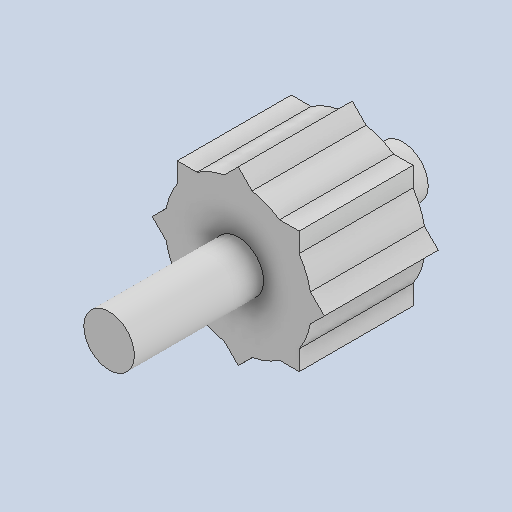
# Autodesk Inventor part: kolo
Saved by Autodesk Inventor 2022.3 (Build 263350000, 350)
## iProperties
Created: 2022-12-14
Part Number: kolo
Material: Generic
Document SubType Name: Modeling
Designer: komputer
Density: 1 g/cm^3
Appearance: Default
Author: komputer
Autodesk Inventor part; units mm, degrees
ref_plane "YZ Plane" through (0, 0, 0) normal (1, 0, 0) x (0, 1, 0)
ref_plane "XZ Plane" through (0, 0, 0) normal (0, 1, 0) x (-1, 0, 0)
ref_plane "XY Plane" through (0, 0, 0) normal (0, 0, 1) x (1, 0, 0)
sketch "Sketch1" plane through (0, 0, 0) normal (0, 0, 1) x (1, 0, 0)
  circle A0 centre (-8.485, -3.042) radius 1.1 projected
  line L0 (-21.0171, 3.396) -> (-20.9715, -5.8039) projected
  line L1 (-19.9666, -6.7989) -> (3.0331, -6.6851) projected
  line L2 (4.0282, -5.6801) -> (3.9826, 3.5198) projected
  circle A1 centre (0, 0) radius 3 projected
  circle A2 centre (-16.9998, -0.0841) radius 3 projected
  circle A3 centre (-8.485, -3.042) radius 1
  line L3 (2.9777, 4.5148) -> (-20.022, 4.401) projected
  arc A4 (-20.9715, -5.8039) -> (-19.9666, -6.7989) centre (-19.9715, -5.7989) ccw projected
  arc A5 (3.0331, -6.6851) -> (4.0282, -5.6801) centre (3.0282, -5.6851) ccw projected
  arc A6 (3.9826, 3.5198) -> (2.9777, 4.5148) centre (2.9826, 3.5148) ccw projected
  arc A7 (-20.022, 4.401) -> (-21.0171, 3.396) centre (-20.0171, 3.401) ccw projected
  point P0 (0, 0)
  dimension "d0" = 2
  constraints: 1 centre point, 1 coincident
  measures "d0" diameter of A3
extrude "Extrusion1" add sketch "Sketch1" against normal blind 5.1 contours A3
sketch "Sketch2" plane through (-8.485, -3.042, -5.1) normal (0, 0, -1) x (-1, 0, 0)
  circle A0 centre (0, 0) radius 1.1 projected
  line L0 (12.5394, 7.938) -> (12.4815, -3.7618) projected
  line L1 (12.4815, -3.7618) -> (-12.5182, -3.6381) projected
  line L2 (-12.5182, -3.6381) -> (-12.4603, 8.0618) projected
  line L3 (-12.4603, 8.0618) -> (12.5394, 7.938) projected
  circle A1 centre (-8.485, 3.042) radius 3 projected
  circle A2 centre (8.5147, 2.9579) radius 3 projected
  line L4 (-0.0183, -3.7) -> (-0.0183, -4.9)
  circle A3 centre (0, 0) radius 4.9
  line L5 (-0.0183, -4.9) -> (-0.0183, -2.9)
  circle A4 centre (0, 0) radius 2.9
  line L6 (0, 2.9) -> (0, 3.4)
  line L7 (0, 3.4) -> (0.5456, 2.8482)
  line L8 (0, 3.4) -> (-0.5456, 2.8482)
  line L9 (-2.4042, 2.4042) -> (-1.6282, 2.3998)
  line L10 (-2.4042, 2.4042) -> (-2.3998, 1.6282)
  line L11 (-3.4, 0) -> (-2.8482, 0.5456)
  line L12 (-3.4, 0) -> (-2.8482, -0.5456)
  line L13 (-2.4042, -2.4042) -> (-2.3998, -1.6282)
  line L14 (-2.4042, -2.4042) -> (-1.6282, -2.3998)
  line L15 (0, -3.4) -> (-0.5456, -2.8482)
  line L16 (0, -3.4) -> (0.5456, -2.8482)
  line L17 (2.4042, -2.4042) -> (1.6282, -2.3998)
  line L18 (2.4042, -2.4042) -> (2.3998, -1.6282)
  line L19 (3.4, 0) -> (2.8482, -0.5456)
  line L20 (3.4, 0) -> (2.8482, 0.5456)
  line L21 (2.4042, 2.4042) -> (2.3998, 1.6282)
  line L22 (2.4042, 2.4042) -> (1.6282, 2.3998)
  line L23 (8.5147, 2.9579) -> (0, 0)
  point P0 (-8.485, 3.042)
  point P1 (2.3998, 1.6282)
  point P2 (-1.6282, 2.3998)
  point P3 (-2.3998, 1.6282)
  point P4 (-2.8482, 0.5456)
  point P5 (-2.8482, -0.5456)
  point P6 (-2.3998, -1.6282)
  point P7 (-1.6282, -2.3998)
  point P8 (-0.5456, -2.8482)
  point P9 (0.5456, -2.8482)
  point P10 (1.6282, -2.3998)
  point P11 (2.8482, -0.5456)
  point P12 (2.8482, 0.5456)
  dimension "d3" = 1.2
  dimension "d4" = 2
  dimension "d5" = 0.5
  dimension "d8" = 360
  constraints: 40 end point, 3 point on circle, 2 coincident, 2 vertical, 1 centre point, 1 midpoint, 1 point on line, 1 symmetric about line, 44 other
  measures "d3" distance of L4.start L4.end
  measures "d4" distance of L4.end L5.end
  measures "d5" distance of L6.start L6.end
extrude "Extrusion2" add sketch "Sketch2" along normal blind 4.5 contours A0 | A4 | L20 L19 A4 | A4 L22 L21 | A4 L6 L7 | L18 L17 A4 | A4 L8 L6 | L15 A4 L5 | L5 A4 L16 L15 | A4 L10 L9 | L14 L13 A4 | A4 L12 L11
sketch "Sketch3" plane through (-8.485, -3.042, -9.6) normal (0, 0, -1) x (-1, 0, 0)
  circle A0 centre (0, 0) radius 1 projected
  point P0 (-8.485, 3.042)
extrude "Extrusion3" add sketch "Sketch3" along normal blind 2
body "Solid1"
